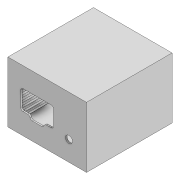
# Autodesk Inventor part: cosmic-watch-enclosure
Saved by Autodesk Inventor 2020 (Build 240168000, 168)
## iProperties
Created: 2020-01-08
Part Number: cosmic-watch-enclosure
Material: Generic
Document SubType Name: Modeling
Designer: kaduo
Density: 1 g/cm^3
Appearance: Default
Author: kaduo
Autodesk Inventor part; units mm, degrees
ref_plane "YZ Plane" through (0, 0, 0) normal (1, 0, 0) x (0, 1, 0)
ref_plane "XZ Plane" through (0, 0, 0) normal (0, 1, 0) x (-1, 0, 0)
ref_plane "XY Plane" through (0, 0, 0) normal (0, 0, 1) x (1, 0, 0)
sketch "Sketch1" plane through (0, 0, 0) normal (0, 0, 1) x (1, 0, 0)
  line L0 (-33.655, -19.939) -> (33.655, -19.939)
  line L1 (33.655, -19.939) -> (33.655, 32.061)
  line L2 (33.655, 32.061) -> (-33.655, 32.061)
  line L3 (-33.655, 32.061) -> (-33.655, -19.939)
  line L4 (-32.258, -18.2118) -> (32.258, -18.2118)
  line L5 (32.258, -18.2118) -> (32.258, 30.1882)
  line L6 (32.258, 30.1882) -> (-32.258, 30.1882)
  line L7 (-32.258, 30.1882) -> (-32.258, -18.2118)
  line L8 (0, 24.1495) -> (0, -29.7749)
  line L9 (-33.655, -15.6718) -> (-29.845, -15.6718)
  line L10 (-29.845, -15.6718) -> (-29.845, -13.8718)
  line L11 (-29.845, -13.8718) -> (-33.655, -13.8718)
  line L12 (-33.655, -13.8718) -> (-33.655, -15.6718)
  line L13 (-33.655, -11.8718) -> (-29.845, -11.8718)
  line L14 (-29.845, -11.8718) -> (-29.845, -10.0718)
  line L15 (-33.655, -10.0718) -> (-33.655, -11.8718)
  line L16 (-29.845, -10.0718) -> (-33.655, -10.0718)
  line L17 (-33.655, -8.0718) -> (-29.845, -8.0718)
  line L18 (-29.845, -8.0718) -> (-29.845, -6.2718)
  line L19 (-33.655, -6.2718) -> (-33.655, -8.0718)
  line L20 (-29.845, -6.2718) -> (-33.655, -6.2718)
  line L21 (-33.655, -4.2718) -> (-29.845, -4.2718)
  line L22 (-29.845, -4.2718) -> (-29.845, -2.4718)
  line L23 (-33.655, -2.4718) -> (-33.655, -4.2718)
  line L24 (-29.845, -2.4718) -> (-33.655, -2.4718)
  line L25 (-33.655, -0.4718) -> (-29.845, -0.4718)
  line L26 (-29.845, -0.4718) -> (-29.845, 1.3282)
  line L27 (-33.655, 1.3282) -> (-33.655, -0.4718)
  line L28 (-29.845, 1.3282) -> (-33.655, 1.3282)
  line L29 (-33.655, 3.3282) -> (-29.845, 3.3282)
  line L30 (-29.845, 3.3282) -> (-29.845, 5.1282)
  line L31 (-33.655, 5.1282) -> (-33.655, 3.3282)
  line L32 (-29.845, 5.1282) -> (-33.655, 5.1282)
  line L33 (-33.655, 7.1282) -> (-29.845, 7.1282)
  line L34 (-29.845, 7.1282) -> (-29.845, 8.9282)
  line L35 (-33.655, 8.9282) -> (-33.655, 7.1282)
  line L36 (-29.845, 8.9282) -> (-33.655, 8.9282)
  line L37 (-33.655, 10.9282) -> (-29.845, 10.9282)
  line L38 (-29.845, 10.9282) -> (-29.845, 12.7282)
  line L39 (-33.655, 12.7282) -> (-33.655, 10.9282)
  line L40 (-29.845, 12.7282) -> (-33.655, 12.7282)
  line L41 (33.655, -15.6718) -> (29.845, -15.6718)
  line L42 (29.845, -15.6718) -> (29.845, -13.8718)
  line L43 (29.845, -13.8718) -> (33.655, -13.8718)
  line L44 (33.655, -13.8718) -> (33.655, -15.6718)
  line L45 (33.655, -11.8718) -> (29.845, -11.8718)
  line L46 (29.845, -11.8718) -> (29.845, -10.0718)
  line L47 (33.655, -10.0718) -> (33.655, -11.8718)
  line L48 (29.845, -10.0718) -> (33.655, -10.0718)
  line L49 (33.655, -8.0718) -> (29.845, -8.0718)
  line L50 (29.845, -8.0718) -> (29.845, -6.2718)
  line L51 (33.655, -6.2718) -> (33.655, -8.0718)
  line L52 (29.845, -6.2718) -> (33.655, -6.2718)
  line L53 (33.655, -4.2718) -> (29.845, -4.2718)
  line L54 (29.845, -4.2718) -> (29.845, -2.4718)
  line L55 (33.655, -2.4718) -> (33.655, -4.2718)
  line L56 (29.845, -2.4718) -> (33.655, -2.4718)
  line L57 (33.655, -0.4718) -> (29.845, -0.4718)
  line L58 (29.845, -0.4718) -> (29.845, 1.3282)
  line L59 (33.655, 1.3282) -> (33.655, -0.4718)
  line L60 (29.845, 1.3282) -> (33.655, 1.3282)
  line L61 (33.655, 3.3282) -> (29.845, 3.3282)
  line L62 (29.845, 3.3282) -> (29.845, 5.1282)
  line L63 (33.655, 5.1282) -> (33.655, 3.3282)
  line L64 (29.845, 5.1282) -> (33.655, 5.1282)
  line L65 (33.655, 7.1282) -> (29.845, 7.1282)
  line L66 (29.845, 7.1282) -> (29.845, 8.9282)
  line L67 (33.655, 8.9282) -> (33.655, 7.1282)
  line L68 (29.845, 8.9282) -> (33.655, 8.9282)
  line L69 (33.655, 10.9282) -> (29.845, 10.9282)
  line L70 (29.845, 10.9282) -> (29.845, 12.7282)
  line L71 (33.655, 12.7282) -> (33.655, 10.9282)
  line L72 (29.845, 12.7282) -> (33.655, 12.7282)
  point P0 (0, 0)
  point P1 (-32.258, -15.6718)
  point P2 (-32.258, -13.8718)
  point P3 (-32.258, -11.8718)
  point P4 (-32.258, -10.0718)
  point P5 (-32.258, -8.0718)
  point P6 (-32.258, -6.2718)
  point P7 (-32.258, -4.2718)
  point P8 (-32.258, -2.4718)
  point P9 (-32.258, -0.4718)
  point P10 (-32.258, 1.3282)
  point P11 (-32.258, 3.3282)
  point P12 (-32.258, 5.1282)
  point P13 (-32.258, 7.1282)
  point P14 (-32.258, 8.9282)
  point P15 (-32.258, 10.9282)
  point P16 (-32.258, 12.7282)
  point P17 (32.258, 12.7282)
  point P18 (32.258, 10.9282)
  point P19 (32.258, 8.9282)
  point P20 (32.258, 7.1282)
  point P21 (32.258, 5.1282)
  point P22 (32.258, 3.3282)
  point P23 (32.258, 1.3282)
  point P24 (32.258, -0.4718)
  point P25 (32.258, -2.4718)
  point P26 (32.258, -4.2718)
  point P27 (32.258, -6.2718)
  point P28 (32.258, -8.0718)
  point P29 (32.258, -10.0718)
  point P30 (32.258, -11.8718)
  point P31 (32.258, -13.8718)
  point P32 (32.258, -15.6718)
  dimension "d0" = 67.31
  dimension "d1" = 52
  dimension "d2" = 64.516
  dimension "d3" = 48.4
  dimension "d32" = 3.81
  dimension "d33" = 1.8
  dimension "d34" = 2.54
  dimension "d37" = 3.8
  constraints: 146 end point, 32 symmetric about line, 6 parallel, 5 horizontal, 3 perpendicular, 2 vertical, 1 point on line, 58 other
  measures "d0" distance of L2.end L1.end
  measures "d1" distance of L1.end L0.end
  measures "d2" distance of L6.end L5.end
  measures "d3" distance of L5.end L4.end
  measures "d32" distance of L11.end L10.end
  measures "d33" distance of L10.end L9.end
  measures "d34" distance between parallel lines of L4 L9
  measures "d37" distance of L9.end L13.end
extrude "Extrusion1" add sketch "Sketch1" along normal blind 72 contours L3 L9 L7 L4 L8 L0 | L8 L4 L5 L41 L1 L0 | L3 L11 L7 L9 | L3 L13 L7 L11 | L7 L11 L10 L9 | L41 L5 L43 L1 | L3 L16 L7 L13 | L43 L5 L45 L1 | L41 L42 L43 L5 | L3 L17 L7 L16 | L7 L16 L14 L13 | L45 L5 L48 L1 | L3 L20 L7 L17 | L48 L5 L49 L1 | L45 L46 L48 L5 | L3 L21 L7 L20 | L7 L20 L18 L17 | L49 L5 L52 L1 | L3 L24 L7 L21 | L52 L5 L53 L1 | L49 L50 L52 L5 | L3 L25 L7 L24 | L7 L24 L22 L21 | L53 L5 L56 L1 | L3 L28 L7 L25 | L56 L5 L57 L1 | L53 L54 L56 L5 | L3 L29 L7 L28 | L7 L28 L26 L25 | L57 L5 L60 L1 | L3 L32 L7 L29 | L60 L5 L61 L1 | L57 L58 L60 L5 | L3 L33 L7 L32 | L7 L32 L30 L29 | L61 L5 L64 L1 | L3 L36 L7 L33 | L64 L5 L65 L1 | L61 L62 L64 L5 | L3 L37 L7 L36 | L7 L36 L34 L33 | L65 L5 L68 L1 | L3 L40 L7 L37 | L68 L5 L69 L1 | L65 L66 L68 L5 | L3 L2 L1 L72 L5 L6 L7 L40 | L7 L40 L38 L37 | L69 L5 L72 L1 | L69 L70 L72 L5
sketch "Sketch2" plane through (0, 0, 72) normal (0, 0, 1) x (1, 0, 0)
  circle A0 centre (18.655, -2.939) radius 3
  line L0 (33.655, 32.061) -> (-33.655, 32.061) projected
  line L1 (33.655, -19.939) -> (33.655, 32.061) projected
  line L2 (-33.655, 32.061) -> (33.655, 32.061)
  line L3 (33.655, 32.061) -> (33.655, -19.939)
  line L4 (33.655, -19.939) -> (-33.655, -19.939)
  line L5 (-33.655, -19.939) -> (-33.655, 32.061)
  line L6 (-22.655, -4.939) -> (5.345, -4.939)
  line L7 (5.345, -4.939) -> (5.345, 15.061)
  line L8 (5.345, 15.061) -> (-22.655, 15.061)
  line L9 (-22.655, 15.061) -> (-22.655, -4.939)
  line L10 (-22.655, -4.939) -> (-14.655, -4.939)
  line L11 (-14.655, -4.939) -> (-14.655, -1.939)
  line L12 (-14.655, -1.939) -> (-22.655, -1.939)
  line L13 (-22.655, -1.939) -> (-22.655, -4.939)
  line L14 (5.345, -4.939) -> (-2.655, -4.939)
  line L15 (-2.655, -4.939) -> (-2.655, -1.939)
  line L16 (-2.655, -1.939) -> (5.345, -1.939)
  line L17 (5.345, -1.939) -> (5.345, -4.939)
  point P0 (0, 0)
  dimension "d42" = 6
  dimension "d46" = 17
  dimension "d47" = 15
  dimension "d48" = 28
  dimension "d49" = 20
  dimension "d50" = 15
  dimension "d51" = 11
  dimension "d81" = 8
  dimension "d82" = 3
  dimension "d83" = 8
  dimension "d84" = 3
  constraints: 32 end point, 8 parallel, 4 horizontal, 4 perpendicular, 1 centre point
  measures "d42" diameter of A0
  measures "d46" distance from line of L4 A0.centre
  measures "d47" distance from line of L1 A0.centre
  measures "d48" distance of L8.end L7.end
  measures "d49" distance of L7.end L6.end
  measures "d50" distance between parallel lines of L4 L6
  measures "d51" distance between parallel lines of L9 L5
  measures "d81" distance of L12.end L11.end
  measures "d82" distance of L11.end L10.end
  measures "d83" distance of L15.end L16.end
  measures "d84" distance of L14.end L15.end
extrude "Extrusion2" add sketch "Sketch2" along normal blind 1.27 contours L1 L4 L5 L0 | L9 L12 L11 L6 | L15 L16 L7 L6
fillet "Fillet2" radius 2 2 edges at (-22.655, 15.061, 72.635) (5.345, 15.061, 72.635)
sketch "Sketch3" plane through (0, 0, 0) normal (0, 0, -1) x (-1, 0, 0)
  line L0 (-33.655, 32.061) -> (33.655, 32.061) projected
  line L1 (-33.655, 32.061) -> (33.655, 32.061)
  line L2 (33.655, 32.061) -> (33.655, -19.939)
  line L3 (33.655, -19.939) -> (-33.655, -19.939)
  line L4 (-33.655, -19.939) -> (-33.655, 32.061)
  line L5 (32.258, 30.1882) -> (-32.258, 30.1882) projected
  line L6 (-32.258, -18.2118) -> (32.258, -18.2118) projected
  line L7 (-32.258, 30.1882) -> (32.258, 30.1882)
  line L8 (32.258, 30.1882) -> (32.258, -18.2118)
  line L9 (32.258, -18.2118) -> (-32.258, -18.2118)
  line L10 (-32.258, -18.2118) -> (-32.258, 30.1882)
  line L11 (-33.655, -19.939) -> (-33.655, 32.061) projected
  line L12 (-33.655, 32.061) -> (-25.655, 32.061)
  line L13 (-25.655, 32.061) -> (-25.655, 24.061)
  line L14 (-25.655, 24.061) -> (-33.655, 24.061)
  line L15 (-33.655, 24.061) -> (-33.655, 32.061)
  line L16 (33.655, -19.939) -> (-33.655, -19.939) projected
  line L17 (-33.655, -19.939) -> (-25.655, -19.939)
  line L18 (-25.655, -19.939) -> (-25.655, -11.939)
  line L19 (-25.655, -11.939) -> (-33.655, -11.939)
  line L20 (-33.655, -11.939) -> (-33.655, -19.939)
  line L21 (33.655, 32.061) -> (25.655, 32.061)
  line L22 (25.655, 32.061) -> (25.655, 24.061)
  line L23 (25.655, 24.061) -> (33.655, 24.061)
  line L24 (33.655, 24.061) -> (33.655, 32.061)
  line L25 (33.655, -19.939) -> (25.655, -19.939)
  line L26 (25.655, -19.939) -> (25.655, -11.939)
  line L27 (25.655, -11.939) -> (33.655, -11.939)
  line L28 (33.655, -11.939) -> (33.655, -19.939)
  point P0 (0, 0)
  point P1 (-32.258, 24.061)
  point P2 (-25.655, 30.1882)
  point P3 (25.655, 30.1882)
  point P4 (32.258, 24.061)
  point P5 (32.258, -11.939)
  point P6 (25.655, -18.2118)
  point P7 (-25.655, -18.2118)
  point P8 (-32.258, -11.939)
  dimension "d54" = 67.31
  dimension "d55" = 52
  dimension "d56" = 64.516
  dimension "d57" = 48.4
  dimension "d58" = 8
  dimension "d59" = 8
  dimension "d60" = 8
  dimension "d61" = 8
  dimension "d62" = 8
  dimension "d63" = 8
  dimension "d64" = 8
  dimension "d65" = 8
  constraints: 48 end point, 12 parallel, 6 horizontal, 6 perpendicular
  measures "d54" distance of L2.end L3.end
  measures "d55" distance of L1.end L2.end
  measures "d56" distance of L6.end L9.end
  measures "d57" distance of L7.end L6.end
  measures "d58" distance of L13.end L14.end
  measures "d59" distance of L12.end L13.end
  measures "d60" distance of L19.end L18.end
  measures "d61" distance of L18.end L17.end
  measures "d62" distance of L23.end L22.end
  measures "d63" distance of L22.end L21.end
  measures "d64" distance of L26.end L27.end
  measures "d65" distance of L25.end L26.end
extrude "Extrusion3" add sketch "Sketch3" against normal blind 4 contours L0 L13 L5 L10 L14 L4 | L0 L22 L5 L13 | L14 L10 L19 L4 | L0 L2 L23 L8 L5 L22 | L13 L14 L10 L5 | L19 L10 L6 L18 L3 L4 | L5 L8 L23 L22 | L19 L18 L6 L10 | L2 L27 L8 L23 | L18 L6 L26 L3 | L2 L3 L26 L6 L8 L27 | L8 L6 L26 L27
sketch "Sketch4" plane through (0, 0, 0) normal (0, 0, -1) x (-1, 0, 0)
  line L0 (33.655, 32.061) -> (33.655, -19.939) projected
  line L1 (-34.036, 25.3037) -> (33.655, 25.3037) construction
  line L2 (-33.655, -19.939) -> (-33.655, 32.061) projected
  line L3 (-33.655, -15.939) -> (33.655, -15.939)
  line L4 (-33.655, 32.061) -> (33.655, 32.061) projected
  line L5 (-29.655, 32.061) -> (-29.655, -19.939)
  line L6 (29.655, 32.061) -> (29.655, -20.7501)
  line L7 (-33.655, 28.061) -> (33.655, 28.061)
  line L8 (33.655, -19.939) -> (-33.655, -19.939) projected
  point P0 (0, 0)
  point P1 (-29.655, 28.061)
  point P2 (29.655, 28.061)
  point P3 (29.655, -15.939)
  point P4 (-29.655, -15.939)
  dimension "d69" = 4
  dimension "d70" = 4
  dimension "d71" = 4
  dimension "d72" = 4
  constraints: 14 point on line, 10 end point, 4 perpendicular, 1 horizontal
  measures "d69" distance between parallel lines of L7 L4
  measures "d70" distance from line of L7.end L6
  measures "d71" distance between parallel lines of L8 L3
  measures "d72" distance from line of L5 L3.start
hole "Hole1" at (29.655, 28.061, 0) at (-29.655, 28.061, 0) at (-29.655, -15.939, 0) at (29.655, -15.939, 0) direction (0, 0, 1) diameter 3.9 depth 4 tip angle 118
fillet "Fillet4" radius 2 6 edges at (-22.655, -1.939, 72.635) (-14.655, -1.939, 72.635) (-14.655, -4.939, 72.635) (5.345, -1.939, 72.635) (-2.655, -1.939, 72.635) (-2.655, -4.939, 72.635)
body "Solid1"
